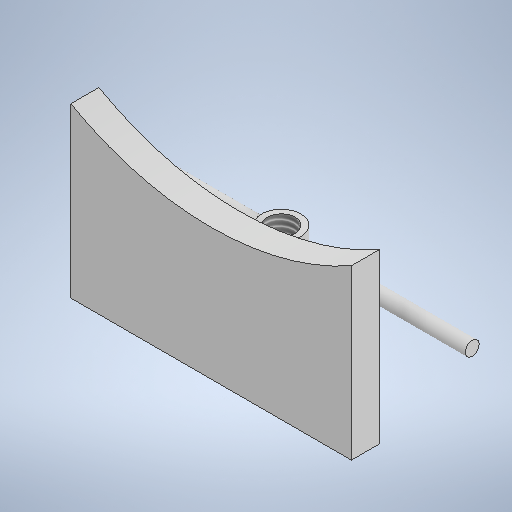
# Autodesk Inventor part: Robot_mouth
Saved by Autodesk Inventor 2025 (Build 290162010, 162A)
## iProperties
Created: 2024-07-17
Part Number: Robot_mouth
Material: Generic
Document SubType Name: Modeling
Designer: saees
Density: 1 g/cm^3
Appearance: Default
Author: saees
Autodesk Inventor part; units mm, degrees
sketch "Sketch1" plane through (0, 0, 0) normal (0, 0, 1) x (1, 0, 0)
  line L0 (-25, 30) -> (-25, 0)
  line L1 (-25, 0) -> (25, 0)
  line L2 (25, 0) -> (25, 30)
  arc A0 (-25, 30) -> (25, 30) centre (0, 74.2226) ccw
  point P0 (0, 0)
  point P1 (0, 0)
  dimension "d0" = 50
  dimension "d1" = 30
  dimension "d2" = 50.8
  constraints: 6 end point, 2 perpendicular, 2 point on circle, 1 centre point, 1 coincident, 1 midpoint, 1 parallel, 1 vertical
  measures "d0" distance of L0.end L1.end
  measures "d1" distance of L1.end L2.end
  measures "d2" radius of A0
extrude "Extrusion1" add sketch "Sketch1" along normal blind 5
sketch "Sketch2" plane through (0, 0, 0) normal (0, 0, -1) x (-1, 0, 0)
  line L0 (-25, 0) -> (-25, 30) projected
  line L1 (25, 30) -> (25, 0) projected
  circle A0 centre (0, 15) radius 2.5
  line L2 (25, 0) -> (-25, 0) projected
  point P0 (0, 0)
  point P1 (25, 15)
  point P2 (0, 0)
  dimension "d5" = 5
  constraints: 2 midpoint, 1 centre point, 1 horizontal alignment, 1 vertical alignment
  measures "d5" diameter of A0
extrude "Extrusion2" add sketch "Sketch2" along normal blind 4
thread "Thread1" size "12-24 UNC" class "2A" standard "ANSI Unified Screw Threads" full length
ref_plane "Work Plane1" through (-25, 15, 0) normal (0, -1, 0) x (1, 0, 0)
sketch "Sketch3" plane through (-25, 15, 0) normal (0, -1, 0) x (1, 0, 0)
  circle A0 centre (25, -7.5) radius 3.5
  circle A1 centre (25, -7.5) radius 2.5
  line L0 (22.5, -4) -> (27.5, -4) projected
  point P0 (25, 0)
  point P1 (25, -4)
  dimension "d11" = 5
  dimension "d12" = 7
  constraints: 2 centre point, 1 coincident, 1 midpoint, 1 tangent, 1 vertical alignment
  measures "d11" diameter of A1
  measures "d12" diameter of A0
extrude "Extrusion3" add sketch "Sketch3" along normal mid plane 5
thread "Thread2" size "12-24 UNC" class "2B" standard "ANSI Unified Screw Threads" full length
sketch "Sketch4" plane through (0, 12.5, -7.5) normal (0, -1, 0) x (1, 0, 0)
  circle A0 centre (0, 0) radius 3.5 projected
  circle A1 centre (0, 0) radius 2.5 projected
  line L0 (0, 3.5) -> (2.5, 3.5) projected
  line L1 (0, 3.5) -> (2.5, 3.5)
  line L2 (2.5, 3.5) -> (2.5, 2.4495)
  line L3 (0, 3.5) -> (-2.5, 3.5)
  line L4 (-2.5, 3.5) -> (-2.5, 2.4495)
  arc A2 (2.5, 2.4495) -> (0, 3.5) centre (0, 0) ccw
  arc A3 (0, 3.5) -> (-2.5, 2.4495) centre (0, 0) ccw
  point P0 (0, 7.5)
  constraints: 8 end point, 6 point on circle, 3 tangent, 2 centre point, 2 concentric, 1 collinear, 1 perpendicular, 1 point on line, 1 vertical
extrude "Extrusion4" add sketch "Sketch4" against normal blind 5 contours A0 L0 L2 | L4 L3 A0
ref_plane "Work Plane2" through (-3.5, 0, 0) normal (-1, 0, 0) x (0, 0, 1)
sketch "Sketch5" plane through (-3.5, 0, 0) normal (-1, 0, 0) x (0, 0, 1)
  line L0 (-5.0505, 17.5) -> (-5.0505, 12.5) projected
  line L1 (-5.0505, 12.5) -> (-5.0505, 12.5) projected
  line L2 (-5.0505, 12.5) -> (-5.0505, 17.5) projected
  line L3 (-5.0505, 17.5) -> (-5.0505, 17.5) projected
  line L4 (-4, 12.5) -> (-4, 15) projected
  line L5 (-4, 15) -> (-4, 12.5) projected
  line L6 (-4, 17.5) -> (-4, 15) projected
  line L7 (-4, 15) -> (-4, 17.5) projected
  line L8 (0, 12.5) -> (0, 17.5) projected
  line L9 (0, 30) -> (0, 0) projected
  line L10 (0, 0) -> (5, 0) projected
  line L11 (5, 30) -> (5, 0) projected
  line L12 (0, 30) -> (5, 30) projected
  line L13 (0, 30) -> (0, 0) projected
  line L14 (-5.0505, 17.5) -> (-11, 17.5) projected
  line L15 (-11, 12.5) -> (-5.0505, 12.5) projected
  circle A0 centre (-8.0253, 15) radius 1.25
  line L16 (-10, 17.5) -> (-5, 17.5) projected
  line L17 (-5, 12.5) -> (-10, 12.5) projected
  dimension "d20" = 2.5
  constraints: 1 centre point
  measures "d20" diameter of A0
extrude "Extrusion5" add sketch "Sketch5" along normal blind 30 contours A0
ref_plane "Work Plane3" through (3.5, 0, 0) normal (1, 0, 0) x (0, 0, -1)
sketch "Sketch6" plane through (3.5, 0, 0) normal (1, 0, 0) x (0, 0, -1)
  line L0 (0, 0) -> (0, 30) projected
  line L1 (4, 12.5) -> (4, 15) projected
  line L2 (4, 15) -> (4, 12.5) projected
  line L3 (4, 17.5) -> (4, 15) projected
  line L4 (4, 15) -> (4, 17.5) projected
  line L5 (0, 17.5) -> (0, 12.5) projected
  line L6 (11, 17.5) -> (5.0505, 17.5) projected
  line L7 (5.0505, 12.5) -> (11, 12.5) projected
  line L8 (11, 17.5) -> (11, 12.5) projected
  line L9 (5.0505, 17.5) -> (5.0505, 12.5) projected
  circle A0 centre (8.0253, 15) radius 1.25
  point P0 (5.0505, 15)
  point P1 (8.0253, 17.5)
  dimension "d24" = 2.5
  constraints: 2 midpoint, 1 centre point, 1 horizontal alignment, 1 vertical alignment
  measures "d24" diameter of A0
extrude "Extrusion6" add sketch "Sketch6" along normal blind 30 contours A0
body "Solid1"
